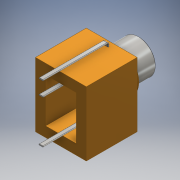
# Autodesk Inventor part: KNOBICONN_TRS
Saved by Autodesk Inventor 2016 (Build 200138000, 138)
## iProperties
Created: 2018-01-09
Part Number: KNOBICONN_TRS
Material: Generic
Document SubType Name: Modeling
Designer: suku
Density: 1 g/cm^3
Appearance: Default
Mass: 0.668688 g
Surface Area: 9.89451 cm^2
Volume: 0.668688 cm^3
Author: suku
Autodesk Inventor part; units mm, degrees
ref_plane "YZ Plane" through (0, 0, 0) normal (1, 0, 0) x (0, 1, 0)
ref_plane "XZ Plane" through (0, 0, 0) normal (0, 1, 0) x (-1, 0, 0)
ref_plane "XY Plane" through (0, 0, 0) normal (0, 0, 1) x (1, 0, 0)
sketch "Sketch1" plane through (0, 0, 0) normal (0, 1, 0) x (-1, 0, 0)
  line L0 (-4.5, 5.7) -> (4.5, 5.7)
  line L1 (4.5, 5.7) -> (4.5, -5.7)
  line L2 (4.5, -5.7) -> (-4.5, -5.7)
  line L3 (-4.5, -5.7) -> (-4.5, 5.7)
  line L4 (-4.5, 5.7) -> (4.5, -5.7) construction
  line L5 (4.5, 5.7) -> (-4.5, -5.7) construction
  point P0 (0, 0)
  dimension "d0" = 9
  dimension "d1" = 11.4
  constraints: 12 end point, 2 midpoint, 2 parallel, 1 horizontal, 1 perpendicular
  measures "d0" distance of L1.end L2.end
  measures "d1" distance of L0.end L1.end
extrude "Extrusion1" add sketch "Sketch1" along normal blind 9
sketch "Sketch2" plane through (0, 0, 0) normal (0, -1, 0) x (1, 0, 0)
  line L0 (4.5, 5.7) -> (-4.5, 5.7) projected
  line L1 (-4.5, 5.7) -> (-4.5, -5.7) projected
  line L2 (-4.5, -5.7) -> (4.5, -5.7) projected
  line L3 (4.5, -5.7) -> (4.5, 5.7) projected
  line L4 (2.71, 3.91) -> (-2.71, 3.91)
  line L5 (-2.71, 3.91) -> (-2.71, -3.91)
  line L6 (-2.71, -3.91) -> (2.71, -3.91)
  line L7 (2.71, -3.91) -> (2.71, 3.91)
  point P0 (0, 0)
  dimension "d4" = 7.82
  constraints: 8 end point, 3 other
  measures "d4" distance between parallel lines of L6 L4
extrude "Extrusion2" cut sketch "Sketch2" against normal blind 7 contours L7 L6 L5 L4
sketch "Sketch4" plane through (0, 9, 0) normal (0, 1, 0) x (1, 0, 0)
  line L0 (0, 0) -> (0, -1.27)
  line L1 (2.5, -4.27) -> (2.5, 1.73)
  line L2 (2.5, 1.73) -> (-2.5, 1.73)
  line L3 (-2.5, 1.73) -> (-2.5, -4.27)
  line L4 (-2.5, -4.27) -> (2.5, -4.27)
  line L5 (2.5, -4.27) -> (-2.5, 1.73) construction
  line L6 (2.5, 1.73) -> (-2.5, -4.27) construction
  arc A0 (-2.5, 1.73) -> (-2.5, -4.27) centre (-0.25, -1.27) ccw
  arc A1 (2.5, -4.27) -> (2.5, 1.73) centre (0.25, -1.27) ccw
  dimension "d17" = 1.27
  dimension "d18" = 6
  dimension "d19" = 5
  dimension "d20" = 3.75
  dimension "d21" = 3.75
  constraints: 14 end point, 4 point on circle, 2 centre point, 2 midpoint, 2 parallel, 2 vertical, 1 perpendicular
  measures "d17" distance of L0.start L0.end
  measures "d18" distance of L1.start L1.end
  measures "d19" distance of L2.end L1.end
  measures "d20" radius of A0
  measures "d21" radius of A1
extrude "Extrusion4" add sketch "Sketch4" along normal blind 0.8
sketch "Sketch5" plane through (0, 9.8, 0) normal (0, 1, 0) x (1, 0, 0)
  arc A0 (2.5, -4.27) -> (2.5, 1.73) centre (0.25, -1.27) ccw projected
  line L0 (2.5, 1.73) -> (-2.5, 1.73) projected
  arc A1 (-2.5, 1.73) -> (-2.5, -4.27) centre (-0.25, -1.27) ccw projected
  line L1 (-2.5, -4.27) -> (2.5, -4.27) projected
  line L2 (0.25, -1.27) -> (-0.25, -1.27)
  circle A2 centre (0, -1.27) radius 3
  circle A3 centre (0, -1.27) radius 2.25
  point P0 (0, 0)
  dimension "d24" = 6
  dimension "d25" = 4.5
  constraints: 2 centre point, 2 end point, 1 coincident, 1 horizontal, 1 midpoint
  measures "d24" diameter of A2
  measures "d25" diameter of A3
extrude "Extrusion5" add sketch "Sketch5" along normal blind 4 separate body contours A2
chamfer "Chamfer1" distance 0.4 angle 45 1 edges at (-2.25, 13.8, 1.27)
chamfer "Chamfer2" distance 0.1 angle 45 1 edges at (-3, 13.8, 1.27)
sketch "Sketch6" plane through (0, 0, 0) normal (1, 0, 0) x (0, 1, 0)
  line L0 (0, 5.7) -> (0, -5.7) projected
  line L1 (8, 6.05) -> (8, 5.7)
  line L2 (8, 5.7) -> (8.2, 5.7)
  line L3 (0, 5.7) -> (9, 5.7) projected
  line L4 (7.8, 6.25) -> (0, 6.25)
  line L5 (0, 6.25) -> (-3.5, 6.25)
  line L6 (-3.5, 6.25) -> (-3.5, 6.45)
  line L7 (-3.5, 6.45) -> (7.8, 6.45)
  line L8 (8, 5.7) -> (8.2, 5.7)
  line L9 (0, 3.91) -> (7, 3.91) projected
  line L10 (0, -3.91) -> (7, -3.91) projected
  line L11 (0, -3.91) -> (0, 3.91) projected
  arc A0 (8, 6.05) -> (7.8, 6.25) centre (7.8, 6.05) ccw
  arc A1 (8.2, 6.05) -> (7.8, 6.45) centre (7.8, 6.05) ccw
  line L12 (8.2, 6.05) -> (8.2, 5.7)
  line L13 (-3.5, -3.91) -> (4.5, -3.91)
  line L14 (4.5, -3.91) -> (4.5, -3.71)
  line L15 (4.5, -3.71) -> (-3.5, -3.71)
  line L16 (0, 3.91) -> (7, 3.91) projected
  line L17 (-3.5, 3.71) -> (4.5, 3.71)
  line L18 (4.5, 3.71) -> (4.5, 3.91)
  line L19 (4.5, 3.91) -> (-3.5, 3.91)
  line L20 (-3.5, 3.91) -> (-3.5, 3.71)
  line L21 (-3.5, -3.91) -> (-3.5, -3.71)
  point P0 (0, 0)
  point P1 (8.2, 6.45)
  point P2 (0, 3.71)
  point P3 (0, -3.71)
  dimension "d37" = 0.2
  dimension "d42" = 3.5
  dimension "d43" = 0.2
  dimension "d44" = 0.2
  dimension "d45" = 0.2
  dimension "d46" = 0.4
  dimension "d49" = 8
  dimension "d50" = 8
  constraints: 32 end point, 8 point on line, 4 perpendicular, 4 point on circle, 3 horizontal, 3 tangent, 3 vertical, 2 centre point, 2 parallel
  measures "d37" distance of L1.end L2.end
  measures "d42" distance of L4.end L5.end
  measures "d43" distance of point (-3.5, 3.91) L17.start
  measures "d44" distance of L13.start point (-3.5, -3.71)
  measures "d45" radius of A0
  measures "d46" radius of A1
  measures "d49" distance of L15.end L14.end
  measures "d50" distance of L19.end L18.end
extrude "Extrusion6" add sketch "Sketch6" along normal mid plane 0.8 separate body
fillet "Fillet1" radius 0.1 20 edges at (-0.4, 0.5, -3.91) (-0.4, 0.5, -3.71) (0.4, 0.5, -3.71) (-0.4, 7.9414, 6.1914) (-0.4, 8, 5.875) (-0.4, 2.15, 6.25) (-0.4, 8.0828, 6.3328) (-0.4, 8.2, 5.875) (-0.4, 2.15, 6.45) (0.4, 8.0828, 6.3328) (0.4, 8.2, 5.875) (0.4, 2.15, 6.45) (-0.4, 0.5, 3.71) (-0.4, 0.5, 3.91) (0.4, 0.5, 3.91) (0.4, 0.5, -3.91) (0.4, 0.5, 3.71) (0.4, 7.9414, 6.1914) (0.4, 8, 5.875) (0.4, 2.15, 6.25)
sketch "Sketch7" plane through (0, 9.8, 1.27) normal (0, 1, 0) x (0, 0, -1)
  circle A0 centre (0, 0) radius 2.25 projected
  point P0 (1.27, 0)
extrude "Extrusion7" cut sketch "Sketch7" against normal through all bodies 1
body "Solid1"
body "Solid2"
body "Solid3"
